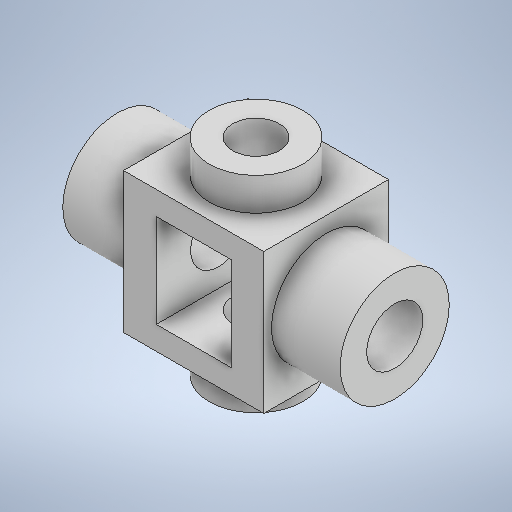
# Autodesk Inventor part: Sólido 1
Saved by Autodesk Inventor 2025 (Build 290162000, 162)
## iProperties
Created: 2024-04-27
Part Number: Sólido 1
Material: Generic
Document SubType Name: Modeling
Designer: kaike
Density: 1 g/cm^3
Appearance: Default
Author: kaike
Autodesk Inventor part; units mm, degrees
ref_plane "YZ Plane" through (0, 0, 0) normal (1, 0, 0) x (0, 1, 0)
ref_plane "XZ Plane" through (0, 0, 0) normal (0, 1, 0) x (-1, 0, 0)
ref_plane "XY Plane" through (0, 0, 0) normal (0, 0, 1) x (1, 0, 0)
sketch "Sketch1" plane through (0, 0, 0) normal (0, 1, 0) x (-1, 0, 0)
  circle A0 centre (0, 0) radius 15
  dimension "d0" = 30
  constraints: 1 centre point, 1 coincident
  measures "d0" diameter of A0
sketch "Sketch2" plane through (0, 0, 0) normal (0, 1, 0) x (-1, 0, 0)
  line L0 (0, 0) -> (22.5, 0)
  line L1 (0, 0) -> (-22.5, 0)
  line L2 (-22.5, 0) -> (-22.5, -20)
  line L3 (-22.5, 0) -> (-22.5, 20)
  line L4 (22.5, 0) -> (22.5, -20)
  line L5 (22.5, -20) -> (-22.5, -20)
  line L6 (22.5, 0) -> (22.5, 20)
  line L7 (22.5, 20) -> (-22.5, 20)
  dimension "d1" = 22.5
  dimension "d2" = 22.5
  dimension "d3" = 20
  dimension "d4" = 20
  constraints: 16 end point, 4 vertical, 2 horizontal, 2 perpendicular
  measures "d1" distance of L0.start L0.end
  measures "d2" distance of L0.start L1.end
  measures "d3" distance of L1.end L2.end
  measures "d4" distance of L1.end L3.end
sketch "Sketch3" plane through (0, 0, 0) normal (0, 1, 0) x (-1, 0, 0)
  circle A0 centre (0, 0) radius 7.5
  dimension "d5" = 15
  constraints: 1 centre point, 1 coincident
  measures "d5" diameter of A0
extrude "Extrusion1" add sketch "Sketch1" along normal mid plane 66
extrude "Extrusion2" add sketch "Sketch2" along normal mid plane 45
extrude "Extrusion3" cut sketch "Sketch3" along normal mid plane 100
sketch "Sketch4" plane through (-22.5, 22.5, 20) normal (0, 0, 1) x (1, 0, 0)
  line L0 (10.5, -22.5) -> (10.5, -37.5)
  line L1 (10.5, -37.5) -> (34.5, -37.5)
  line L2 (34.5, -37.5) -> (34.5, -22.5)
  line L3 (10.5, -22.5) -> (10.5, -7.5)
  line L4 (10.5, -7.5) -> (34.5, -7.5)
  line L5 (34.5, -7.5) -> (34.5, -22.5)
  point P0 (22.5, -22.5)
  dimension "d14" = 15
  constraints: 12 end point, 2 perpendicular
  measures "d14" distance of L0.start L0.end
sketch "Sketch5" plane through (22.5, -22.5, -20) normal (1, 0, 0) x (0, 0, -1)
  circle A0 centre (-20, 22.5) radius 17.5
  dimension "d15" = 35
  constraints: 1 centre point, 1 coincident
  measures "d15" diameter of A0
sketch "Sketch6" plane through (22.5, -22.5, -20) normal (1, 0, 0) x (0, 0, -1)
  circle A0 centre (-20, 22.5) radius 9
  dimension "d28" = 18
  constraints: 1 centre point, 1 coincident
  measures "d28" diameter of A0
extrude "Extrusion4" add sketch "Sketch5" along normal blind 22
sketch "Sketch7" plane through (-22.5, -22.5, 20) normal (-1, 0, 0) x (0, 0, 1)
  circle A0 centre (-20, 22.5) radius 17.5
  dimension "d20" = 35
  constraints: 1 centre point, 1 coincident
  measures "d20" diameter of A0
extrude "Extrusion5" add sketch "Sketch7" along normal blind 22
extrude "Extrusion6" cut sketch "Sketch4" against normal blind 100
extrude "Extrusion7" cut sketch "Sketch6" along normal mid plane 200
body "Solid1"
